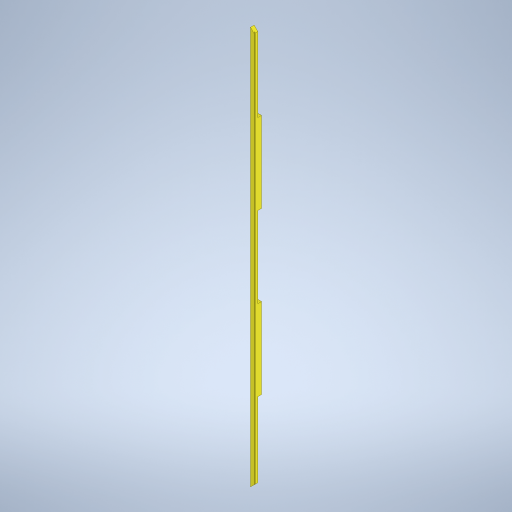
# Autodesk Inventor part: Frame Side(Long)
Saved by Autodesk Inventor 2024 (Build 280153000, 153)
## iProperties
Created: 2024-02-22
Part Number: Frame Side(Long)
Material: Generic
Document SubType Name: Modeling
Designer: flynf
Density: 1 g/cm^3
Appearance: Canary
Author: flynf
Autodesk Inventor part; units mm, degrees
ref_plane "YZ Plane" through (0, 0, 0) normal (1, 0, 0) x (0, 1, 0)
ref_plane "XZ Plane" through (0, 0, 0) normal (0, 1, 0) x (-1, 0, 0)
ref_plane "XY Plane" through (0, 0, 0) normal (0, 0, 1) x (1, 0, 0)
sketch "Sketch1" plane through (0, 0, 0) normal (1, 0, 0) x (0, 1, 0)
  line L0 (0, 0) -> (2070.1, 0)
  line L1 (2070.1, 0) -> (2070.1, -19.05)
  line L2 (2070.1, -19.05) -> (0, -19.05)
  line L3 (0, -19.05) -> (0, 0)
  line L4 (1244.6, -19.05) -> (1244.6, -38.1)
  line L5 (1244.6, -38.1) -> (1663.7, -38.1)
  line L6 (1663.7, -38.1) -> (1663.7, -19.05)
  line L7 (825.5, -19.05) -> (406.4, -19.05)
  line L8 (406.4, -19.05) -> (406.4, -38.1)
  line L9 (406.4, -38.1) -> (825.5, -38.1)
  line L10 (825.5, -38.1) -> (825.5, -19.05)
  dimension "d0" = 2070.1
  dimension "d1" = 19.05
  dimension "d2" = 19.05
  dimension "d3" = 419.1
  dimension "d4" = 406.4
  dimension "d20" = 19.05
  dimension "d21" = 419.1
  dimension "d22" = 419.1
  constraints: 22 end point, 4 parallel, 4 perpendicular, 3 point on line, 2 horizontal, 1 vertical
  measures "d0" distance of L1.end L2.end
  measures "d1" distance of L0.end L1.end
  measures "d2" distance of L4.start L4.end
  measures "d3" distance of L4.end L5.end
  measures "d4" distance between parallel lines of L1 L6
  measures "d20" distance of L9.end L7.start
  measures "d21" distance between parallel lines of L10 L4
  measures "d22" distance of L8.end L9.end
extrude "Extrusion1" add sketch "Sketch1" along normal blind 19.05
sketch "Sketch2" plane through (19.05, 0, 0) normal (1, 0, 0) x (0, 0, -1)
  line L0 (19.05, 2070.1) -> (0, 2070.1) projected
  line L1 (0, 0) -> (19.05, 0) projected
  line L2 (3.175, 2070.1) -> (6.35, 2070.1)
  line L3 (6.35, 2070.1) -> (6.35, 0)
  line L4 (6.35, 0) -> (3.175, 0)
  line L5 (3.175, 0) -> (3.175, 2070.1)
  line L6 (0, 2070.1) -> (0, 0) projected
  dimension "d7" = 3.175
  dimension "d8" = 3.175
  constraints: 8 end point, 2 parallel, 2 point on line, 1 horizontal, 1 perpendicular
  measures "d7" distance between parallel lines of L5 L3
  measures "d8" distance between parallel lines of L6 L5
extrude "Extrusion2" cut sketch "Sketch2" against normal blind 3.175 contours L3 L1 L5 L0
sketch "Sketch3" plane through (0, 0, 0) normal (0, 0, 1) x (1, 0, 0)
  line L0 (0, 0) -> (19.05, 19.05)
  line L1 (19.05, 2070.1) -> (19.05, 0) projected
  line L2 (0, 0) -> (26.9408, 0) construction
  line L3 (0, 1054.1) -> (19.05, 1035.05)
  line L4 (0, 1054.1) -> (26.9408, 1054.1) construction
  dimension "d11" = 45
  dimension "d12" = 45
  constraints: 8 end point, 2 equal length, 2 horizontal, 1 midpoint, 1 point on line
  measures "d11" angle of L2 L0
  measures "d12" angle of L3 L4
extrude "Extrusion3" cut sketch "Sketch3" against normal through all fills toward (9.5604, 9.4896) open curves L0
sketch "Sketch4" plane through (0, 0, 0) normal (0, 0, 1) x (1, 0, 0)
  line L0 (0, 1663.7) -> (0, 2070.1) projected
  line L1 (0, 2070.1) -> (19.05, 2051.05)
  line L2 (19.05, 2070.1) -> (19.05, 19.05) projected
  line L3 (0, 2070.1) -> (26.9408, 2070.1) construction
  point P0 (0, 0)
  dimension "d16" = 45
  constraints: 4 end point, 1 equal length, 1 horizontal, 1 point on line
  measures "d16" angle of L1 L3
extrude "Extrusion4" cut sketch "Sketch4" against normal through all fills toward (9.5604, 2060.6104) open curves L1
body "Solid1"
